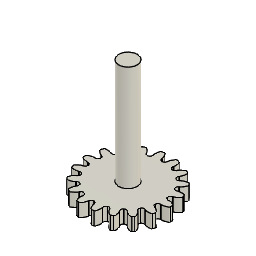
Main-Gear (Autodesk Fusion 360 design; units mm, degrees)
description: Spur Gear; Module: 1.6666666; Num Teeth: 18; Pressure Angle: 20.0; Backlash: 0.00 mm
Autodesk Fusion 360 part; units mm, degrees
sketch "Esboço1" plane through (0, 0, 0) normal (0, 0, 1) x (1, 0, 0) in component "Spur Gear (18 teeth)"
  circle A0 centre (0, 0) radius 12.9492
  circle A1 centre (0, 0) radius 3.5
  dimension "d21_1" = 7
  measures "d21_1" diameter of A1
extrude "Extrusão1" add sketch "Esboço1" along normal blind 5 in component "Spur Gear (18 teeth)"
sketch "Esboço2" plane through (0, 0, 0) normal (0, 0, 1) x (1, 0, 0) in component "Spur Gear (18 teeth)"
  spline S0 degree 5 poles (14.0219, -1.4376) (14.0294, -1.4384) (14.0444, -1.4397) (14.067, -1.4411) (14.0972, -1.4417) (14.1349, -1.441) (14.1728, -1.439) (14.2106, -1.4364) (14.2485, -1.4333) (14.2865, -1.43) (14.3244, -1.4263) (14.3624, -1.4224) (14.4004, -1.4179) (14.4384, -1.4129) (14.4764, -1.4073) (14.5144, -1.4012) (14.5524, -1.3946) (14.5905, -1.3876) (14.6285, -1.3804) (14.6665, -1.3728) (14.7046, -1.3648) (14.7426, -1.3566) (14.7806, -1.348) (14.8186, -1.3391) (14.8567, -1.3298) (14.8947, -1.3201) (14.9327, -1.3102) (14.9707, -1.2999) (15.0087, -1.2893) (15.0466, -1.2785) (15.0846, -1.2673) (15.1225, -1.2559) (15.1604, -1.2441) (15.1983, -1.2321) (15.2361, -1.2198) (15.274, -1.2072) (15.3119, -1.1944) (15.3498, -1.1813) (15.3876, -1.168) (15.4255, -1.1544) (15.4632, -1.1405) (15.5009, -1.1263) (15.5385, -1.1117) (15.5761, -1.0968) (15.6136, -1.0817) (15.6513, -1.0665) (15.689, -1.0512) (15.7268, -1.0359) (15.7647, -1.0205) (15.8025, -1.0047) (15.8401, -0.9883) (15.8773, -0.9713) (15.9141, -0.9536) (15.9507, -0.9354) (15.9874, -0.9172) (16.0245, -0.8994) (16.0624, -0.8824) (16.1011, -0.8663) (16.1403, -0.8507) (16.1794, -0.8346) (16.2174, -0.817) (16.2534, -0.7966) (16.2866, -0.7724) (16.3164, -0.744) (16.3427, -0.7116) (16.3654, -0.6757) (16.385, -0.6373) (16.4017, -0.5974) (16.4159, -0.5568) (16.4278, -0.5162) (16.4376, -0.4758) (16.4438, -0.4438) (16.4475, -0.42) (16.4495, -0.4043) (16.4504, -0.3964) knots 0 0 0 0 0 0 0.01428571 0.02857143 0.04285714 0.05714286 0.07142857 0.08571429 0.1 0.11428571 0.12857143 0.14285714 0.15714286 0.17142857 0.18571429 0.2 0.21428571 0.22857143 0.24285714 0.25714286 0.27142857 0.28571429 0.3 0.31428571 0.32857143 0.34285714 0.35714286 0.37142857 0.38571429 0.4 0.41428571 0.42857143 0.44285714 0.45714286 0.47142857 0.48571429 0.5 0.51428571 0.52857143 0.54285714 0.55714286 0.57142857 0.58571429 0.6 0.61428571 0.62857143 0.64285714 0.65714286 0.67142857 0.68571429 0.7 0.71428571 0.72857143 0.74285714 0.75714286 0.77142857 0.78571429 0.8 0.81428571 0.82857143 0.84285714 0.85714286 0.87142857 0.88571429 0.9 0.91428571 0.92857143 0.94285714 0.95714286 0.97142857 0.98571429 1 1 1 1 1 1
  spline S1 degree 5 poles (14.0219, 1.4376) (14.0294, 1.4384) (14.0444, 1.4397) (14.067, 1.4411) (14.0972, 1.4417) (14.1349, 1.441) (14.1728, 1.439) (14.2106, 1.4364) (14.2485, 1.4333) (14.2865, 1.43) (14.3244, 1.4263) (14.3624, 1.4224) (14.4004, 1.4179) (14.4384, 1.4129) (14.4764, 1.4073) (14.5144, 1.4012) (14.5524, 1.3946) (14.5905, 1.3876) (14.6285, 1.3804) (14.6665, 1.3728) (14.7046, 1.3648) (14.7426, 1.3566) (14.7806, 1.348) (14.8186, 1.3391) (14.8567, 1.3298) (14.8947, 1.3201) (14.9327, 1.3102) (14.9707, 1.2999) (15.0087, 1.2893) (15.0466, 1.2785) (15.0846, 1.2673) (15.1225, 1.2559) (15.1604, 1.2441) (15.1983, 1.2321) (15.2361, 1.2198) (15.274, 1.2072) (15.3119, 1.1944) (15.3498, 1.1813) (15.3876, 1.168) (15.4255, 1.1544) (15.4632, 1.1405) (15.5009, 1.1263) (15.5385, 1.1117) (15.5761, 1.0968) (15.6136, 1.0817) (15.6513, 1.0665) (15.689, 1.0512) (15.7268, 1.0359) (15.7647, 1.0205) (15.8025, 1.0047) (15.8401, 0.9883) (15.8773, 0.9713) (15.9141, 0.9536) (15.9507, 0.9354) (15.9874, 0.9172) (16.0245, 0.8994) (16.0624, 0.8824) (16.1011, 0.8663) (16.1403, 0.8507) (16.1794, 0.8346) (16.2174, 0.817) (16.2534, 0.7966) (16.2866, 0.7724) (16.3164, 0.744) (16.3427, 0.7116) (16.3654, 0.6757) (16.385, 0.6373) (16.4017, 0.5974) (16.4159, 0.5568) (16.4278, 0.5162) (16.4376, 0.4758) (16.4438, 0.4438) (16.4475, 0.42) (16.4495, 0.4043) (16.4504, 0.3964) knots 0 0 0 0 0 0 0.01428571 0.02857143 0.04285714 0.05714286 0.07142857 0.08571429 0.1 0.11428571 0.12857143 0.14285714 0.15714286 0.17142857 0.18571429 0.2 0.21428571 0.22857143 0.24285714 0.25714286 0.27142857 0.28571429 0.3 0.31428571 0.32857143 0.34285714 0.35714286 0.37142857 0.38571429 0.4 0.41428571 0.42857143 0.44285714 0.45714286 0.47142857 0.48571429 0.5 0.51428571 0.52857143 0.54285714 0.55714286 0.57142857 0.58571429 0.6 0.61428571 0.62857143 0.64285714 0.65714286 0.67142857 0.68571429 0.7 0.71428571 0.72857143 0.74285714 0.75714286 0.77142857 0.78571429 0.8 0.81428571 0.82857143 0.84285714 0.85714286 0.87142857 0.88571429 0.9 0.91428571 0.92857143 0.94285714 0.95714286 0.97142857 0.98571429 1 1 1 1 1 1
  arc A0 (16.4504, -0.3964) -> (16.4504, 0.3964) centre (-0.0983, 0) ccw
  line L0 (12.8717, -1.3207) -> (14.0219, -1.4376)
  line L1 (12.8717, 1.3207) -> (14.0219, 1.4376)
  line L2 (12.8717, -1.3207) -> (12.8717, 1.3207)
  point P0 (14.2066, -1.4366)
  point P1 (14.393, -1.4187)
  point P2 (14.5803, -1.3894)
  point P3 (14.7684, -1.3507)
  point P4 (14.957, -1.3035)
  point P5 (15.146, -1.2486)
  point P6 (15.3352, -1.1863)
  point P7 (15.5246, -1.1171)
  point P8 (15.7139, -1.0411)
  point P9 (15.9031, -0.9588)
  point P10 (16.0922, -0.8701)
  point P11 (16.2809, -0.7754)
  point P12 (16.4, -0.6)
  point P13 (14.2066, 1.4366)
  point P14 (14.393, 1.4187)
  point P15 (14.5803, 1.3894)
  point P16 (14.7684, 1.3507)
  point P17 (14.957, 1.3035)
  point P18 (15.146, 1.2486)
  point P19 (15.3352, 1.1863)
  point P20 (15.5246, 1.1171)
  point P21 (15.7139, 1.0411)
  point P22 (15.9031, 0.9588)
  point P23 (16.0922, 0.8701)
  point P24 (16.2809, 0.7754)
  point P25 (16.4, 0.6)
extrude "Extrusão2" add sketch "Esboço2" along normal blind 5 in component "Spur Gear (18 teeth)"
fillet "Arredondamento1" radius 0.98 2 edges at (12.8816, -1.3217, 2.5) (12.8816, 1.3217, 2.5) in component "Spur Gear (18 teeth)"
pattern_circular "Padrão circular1" count 18 over 360 about axis through (0, 0, 0) along (0, 0, 1) of "Extrusão2", "Arredondamento1" in component "Spur Gear (18 teeth)"
sketch "Esboço3" plane through (0, 0, 0) normal (0, 0, 1) x (1, 0, 0) in component "Spur Gear (18 teeth)"
  circle A0 centre (0, 0) radius 15 construction
extrude "Extrusão4" add sketch "Esboço1" along normal blind 45 contours A1 in component "Spur Gear (18 teeth)"
extrude "Extrusão5" [suppressed] in component "Spur Gear (18 teeth)"
extrude "Extrusão3" [suppressed] in component "Spur Gear (18 teeth)"
component "Spur Gear (18 teeth)" placed x (1, 0, 0) y (0, 1, 0) z (0, 0, 1) at (0, 0, 0)
